Autodesk Inventor part; units mm, degrees
(part 3 of 3)
sketch "Sketch20" plane through (-4.2986, 24.5, 27.7) normal (0, -1, 0) x (1, 0, 0)
  arc A0 (20.8845, -2.8543) -> (23.789, -26.7) centre (29.9486, -13.85) ccw projected
  line L0 (23.789, -27.7) -> (23.789, -26.7) projected
  line L1 (43.7986, -27.7) -> (23.789, -27.7) projected
  line L2 (43.7986, 0) -> (43.7986, -27.7) projected
  line L3 (39.4105, 0) -> (43.7986, 0) projected
  line L4 (39.4105, -21.7089) -> (39.4105, 0) projected
  arc A1 (35.8615, -24.6355) -> (39.4105, -21.7089) centre (29.9486, -13.85) ccw projected
  line L5 (32.1777, -20.1683) -> (35.8615, -24.6355) projected
  line L6 (31.5107, -19.0191) -> (32.1777, -20.1683) projected
  arc A2 (24.5486, -13.85) -> (31.5107, -19.0191) centre (29.9486, -13.85) ccw projected
  line L7 (24.1705, -10.4583) -> (24.5486, -13.85) projected
  arc A3 (5.8313, -6.9369) -> (7.5647, -12.9022) centre (13.5164, -7.9382) ccw projected
  line L8 (20.8845, -2.8543) -> (20.8845, -5.5354) projected
  line L9 (43.7986, 0) -> (36.7986, 0)
  line L10 (36.7986, 0) -> (36.7986, -6)
  line L11 (36.7986, -6) -> (43.7986, -6)
  line L12 (43.7986, -6) -> (43.7986, 0)
  arc A4 (27.7194, -7.5317) -> (24.1705, -10.4583) centre (29.9486, -13.85) ccw projected
  line L13 (24.0356, -3.0645) -> (27.7194, -7.5317) projected
  arc A5 (24.0356, -3.0645) -> (20.8845, -5.5354) centre (29.9486, -13.85) ccw projected
  arc A6 (7.5647, -12.9022) -> (7.4306, -12.3314) centre (2.2486, -13.85) ccw projected
  arc A7 (7.4306, -12.3314) -> (10.4371, -0.8262) centre (5.0916, -5.5748) ccw projected
  arc A8 (5.8313, -6.9369) -> (6.4319, -4.7962) centre (5.0916, -5.5748) ccw projected
  arc A9 (10.4371, -0.8262) -> (6.4319, -4.7962) centre (13.5164, -7.9382) ccw projected
  point P0 (4.2986, -27.7)
  point P1 (39.4105, -6)
  dimension "d109" = 7
  dimension "d110" = 6
  constraints: 8 end point, 2 parallel, 1 horizontal, 1 perpendicular
  measures "d109" distance of L11.end L10.end
  measures "d110" distance of L10.end L9.end
extrude "Extrusion17" add sketch "Sketch20" along normal up to surface (3.3 mm away) contours L11 L10 L9 L4
fillet "Fillet1" radius 2 1 edges at (32.5, 22.85, 21.7)
sketch "Sketch21" plane through (39.5, 21.2, 27.7) normal (1, 0, 0) x (0, 0, -1)
  line L0 (6, 0) -> (6, 3.3) projected
  line L1 (0, 0) -> (0, 8.6) projected
  line L2 (6, 3.3) -> (6, 8.6)
  line L3 (0, 0) -> (27.7, 0) projected
  line L4 (0, 0) -> (6, 8.6)
  line L5 (0, 8.6) -> (6, 0)
  point P0 (27.7, -21.2)
  point P1 (3, 4.3)
  point P2 (0, 5.4)
  constraints: 6 end point, 1 midpoint, 1 vertical
hole "Hole5" at (39.5, 25.5, 24.7) direction (-1, 0, 0) diameter 4 depth 6.5 counterbore diameter 5 counterbore depth 1.5
sketch "Sketch22" plane through (-4.2986, 29.8, 27.7) normal (0, 1, 0) x (1, 0, 0)
  line L0 (43.7986, 27.7) -> (38.252, 27.7) projected
  arc A0 (38.252, 27.7) -> (18.7451, 27.7) centre (28.4986, 22.8337) ccw projected
  arc A1 (12.752, 27.7) -> (-6.7549, 27.7) centre (2.9986, 22.8337) ccw projected
  line L1 (-6.7549, 27.7) -> (-10.0014, 27.7) projected
  line L2 (-10.0014, 27.7) -> (-10.0014, 0) projected
  line L3 (10.1832, 0) -> (43.7986, 0) projected
  arc A2 (0, 0) -> (10.1832, 0) centre (5.0916, 5.5748) ccw projected
  line L4 (-10.0014, 0) -> (0, 0) projected
  line L5 (43.7986, 0) -> (43.7986, 27.7) projected
  circle A3 centre (-6.5014, 3.5) radius 3.5
  line L6 (-10.0014, 27.7) -> (-10.0014, 0) projected
  circle A4 centre (40.2986, 14.5803) radius 3.5
  circle A5 centre (24.0333, 9.1435) radius 3.5
  circle A6 centre (-6.5014, 12.012) radius 3.5
  line L7 (18.7451, 27.7) -> (12.752, 27.7) projected
  dimension "d123" = 7
  dimension "d125" = 7
  dimension "d127" = 7
  dimension "d135" = 7
  constraints: 7 tangent, 4 centre point, 4 coincident
  measures "d123" diameter of A3
  measures "d125" diameter of A4
  measures "d127" diameter of A5
  measures "d135" diameter of A6
hole "Hole6" at (-10.8, 29.8, 24.2) at (36, 29.8, 13.1197) at (19.7348, 29.8, 18.5565) at (-10.8, 29.8, 15.688) direction (0, -1, 0) diameter 4 depth 4 counterbore diameter 5 counterbore depth 1
sketch "Sketch23" plane through (-14.3, 16.2, 27.7) normal (0, 0, 1) x (1, 0, 0)
  line L0 (20.1847, 0) -> (20.1847, 13.6) projected
  line L1 (20.1847, 0) -> (33.7905, 0) projected
  line L2 (33.7905, 0) -> (33.7905, 8.3) projected
  line L3 (0, 0) -> (0, 13.6) projected
  line L4 (0, 0) -> (10.0014, 0) projected
  line L5 (10.0014, 0) -> (10.0014, 13.6) projected
  line L6 (0, 0) -> (0, 5.7) projected
  line L7 (0, 0) -> (6, 0)
  line L8 (6, 0) -> (6, 6)
  line L9 (6, 6) -> (0, 6)
  line L10 (0, 6) -> (0, 0)
  line L11 (0, 6) -> (6, 0)
  line L12 (33.7905, 0) -> (0, 0) projected
  line L13 (0, 0) -> (6, 6)
  line L14 (25.7, 6) -> (25.7, 0)
  line L15 (25.7, 5) -> (25.7, 0) projected
  line L16 (30.7, 6) -> (30.7, 0)
  line L17 (30.7, 6) -> (25.7, 0)
  line L18 (20.1847, 0) -> (20.1847, 13.6) projected
  line L19 (20.1847, 0) -> (33.7905, 0) projected
  line L20 (33.7905, 0) -> (33.7905, 8.3) projected
  line L21 (0, 0) -> (0, 13.6) projected
  line L22 (0, 0) -> (10.0014, 0) projected
  line L23 (10.0014, 0) -> (10.0014, 13.6) projected
  line L24 (33.7905, 8.3) -> (46.8, 8.3) projected
  line L25 (53.8, 5) -> (46.8, 5) projected
  line L26 (53.8, 5) -> (53.8, 13.6) projected
  line L27 (33.7905, 8.3) -> (46.8, 8.3) projected
  line L28 (53.8, 5) -> (46.8, 5) projected
  line L29 (53.8, 5) -> (53.8, 13.6) projected
  line L30 (0, 13.6) -> (10.0014, 13.6) projected
  line L31 (20.1847, 13.6) -> (53.8, 13.6) projected
  line L32 (0, 13.6) -> (10.0014, 13.6) projected
  line L33 (20.1847, 13.6) -> (53.8, 13.6) projected
  line L34 (46.8, 8.3) -> (46.8, 5) projected
  line L35 (46.8, 8.3) -> (46.8, 5) projected
  point P0 (14.3, -16.2)
  point P1 (0, 13.6)
  point P2 (3, 3)
  point P3 (30.8859, 5)
  point P4 (28.2, 3)
  dimension "d136" = 6
  dimension "d137" = 6
  dimension "d138" = 5
  dimension "d146" = 1
  dimension "d147" = 0
  constraints: 18 end point, 3 point on line, 2 midpoint, 2 parallel, 2 perpendicular, 1 horizontal
  measures "d136" distance of L9.end L8.end
  measures "d137" distance of L8.end L7.end
  measures "d138" distance between parallel lines of L15 L16
  measures "d146" vertical distance of L16.start point (30.886, 5)
  measures "d147" vertical distance of L14.start L16.start
hole "Hole7" at (-11.3, 19.2, 27.7) at (13.9, 19.2, 27.7) direction (0, 0, -1) diameter 3 depth 3.5 counterbore diameter 5 counterbore depth 0.5
body "Solid1"
